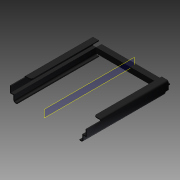
# Autodesk Inventor part: battery rails
Saved by Autodesk Inventor 2012 (Build 160160000, 160)
## iProperties
Created: 2012-03-07
Part Number: battery rails
Material: Default
Document SubType Name: Modeling
Designer: esv
Density: 1 g/cm^3
Author: esv
Autodesk Inventor part; units mm, degrees
ref_plane "YZ Plane" through (0, 0, 0) normal (1, 0, 0) x (0, 1, 0)
ref_plane "XZ Plane" through (0, 0, 0) normal (0, 1, 0) x (-1, 0, 0)
ref_plane "XY Plane" through (0, 0, 0) normal (0, 0, 1) x (1, 0, 0)
sketch "Sketch1" plane through (0, 0, 0) normal (0, 0, 1) x (1, 0, 0)
  line L0 (0, 31.75) -> (4.1656, 31.75)
  line L1 (4.1656, 31.75) -> (4.1656, 0)
  line L2 (4.1656, 0) -> (0, 0)
  line L3 (0, 0) -> (0, 31.75)
  line L4 (4.1656, 0) -> (14.8844, 0)
  line L5 (14.8844, 0) -> (14.8844, 4.1656)
  line L6 (14.8844, 4.1656) -> (4.1656, 4.1656)
  line L7 (4.1656, 4.1656) -> (4.1656, 0)
  line L8 (14.8844, 4.1656) -> (19.05, 4.1656)
  line L9 (19.05, 4.1656) -> (19.05, -17.161)
  line L10 (19.05, -17.161) -> (14.8844, -17.161)
  line L11 (14.8844, -17.161) -> (14.8844, 4.1656)
  arc A0 (14.8844, -17.161) -> (33.9344, -26.2503) centre (26.5778, -17.161) ccw
  arc A1 (19.05, -17.161) -> (31.3137, -23.0124) centre (26.5778, -17.161) ccw
  line L12 (33.9344, -26.2503) -> (31.3137, -23.0124)
  line L13 (16.255, -28.8544) -> (45.3124, -28.8544)
  dimension "d0" = 31.75
  dimension "d1" = 19.05
  dimension "d2" = 4.1656
  dimension "d5" = 33.02
  dimension "d6" = 19.05
  dimension "d7" = 5.842
  constraints: 28 end point, 6 parallel, 4 perpendicular, 4 point on circle, 3 equal length, 3 horizontal, 2 centre point, 2 tangent, 1 coincident, 1 concentric
  measures "d0" distance of L2.end L0.start
  measures "d1" distance between parallel lines of L3 L9
  measures "d2" distance of L0.start L0.end
  measures "d5" distance between parallel lines of L8 L13
  measures "d6" distance from line of L11 L12.start
  measures "d7" distance from line of L13 L12.end
extrude "Extrusion1" add sketch "Sketch1" along normal blind 381
sketch "Sketch2" plane through (0, 0, 0) normal (0, 0, -1) x (-1, 0, 0)
  line L0 (0, 31.75) -> (0, 0) projected
  line L1 (-4.1656, 31.75) -> (0, 31.75) projected
  line L2 (-4.1656, 4.1656) -> (-4.1656, 31.75) projected
  arc A0 (-33.9344, -26.2503) -> (-14.8844, -17.161) centre (-26.5778, -17.161) ccw projected
  line L3 (-31.75, 38.5572) -> (-6.8072, 38.5572)
  line L4 (-6.8072, 38.5572) -> (-6.8072, 34.3916)
  line L5 (-6.8072, 34.3916) -> (-31.75, 34.3916)
  line L6 (-31.75, 34.3916) -> (-31.75, 38.5572)
  arc A1 (0, 31.75) -> (-6.8072, 38.5572) centre (-6.8072, 31.75) ccw
  arc A2 (-4.1656, 31.75) -> (-6.8072, 34.3916) centre (-6.8072, 31.75) ccw
  line L7 (-19.05, -28.8544) -> (-58.4387, -28.8544)
  dimension "d12" = 67.4116
  dimension "d13" = 31.75
  constraints: 10 end point, 4 point on circle, 4 tangent, 2 centre point, 2 parallel, 2 perpendicular, 1 concentric, 1 horizontal
  measures "d12" distance between parallel lines of L3 L7
  measures "d13" distance between parallel lines of L0 L6
extrude "Extrusion2" add sketch "Sketch2" against normal blind 314.325
fillet "Fillet1" radius 9.525 1 edges at (31.75, 36.4744, 314.325)
ref_plane "Work Plane1" through (177.8, 0, 381) normal (-1, 0, 0) x (0, 0, 1)
mirror "Mirror1" about plane through (177.8, 0, 381) normal (-1, 0, 0) of "Extrusion1", "Extrusion2", "Fillet1"
sketch "Sketch3" plane through (19.05, -17.161, 0) normal (1, 0, 0) x (0, 0, -1)
  line L0 (0, 0) -> (0, 21.3266)
  line L1 (0, 21.3266) -> (-381, 21.3266) projected
  line L2 (0, -4.0734) -> (5.08, -4.0734)
  line L3 (5.08, -4.0734) -> (5.08, 21.3266)
  line L4 (5.08, 21.3266) -> (0, 21.3266)
  line L5 (0, 21.3266) -> (0, -4.0734)
  line L6 (5.08, 21.3266) -> (25.4, 21.3266)
  line L7 (25.4, 21.3266) -> (25.4, 16.2466)
  line L8 (25.4, 16.2466) -> (5.08, 16.2466)
  line L9 (5.08, 16.2466) -> (5.08, 21.3266)
  point P0 (0, 17.161)
  dimension "d18" = 5.08
  dimension "d19" = 25.4
  dimension "d20" = 25.4
  constraints: 18 end point, 4 parallel, 3 perpendicular, 2 horizontal, 1 collinear
  measures "d18" distance of L6.end L7.end
  measures "d19" distance between parallel lines of L7 L5
  measures "d20" distance between parallel lines of L2 L4
extrude "crosspiece" add sketch "Sketch3" along normal up to surface (317.5 mm away)
body "Solid1"
